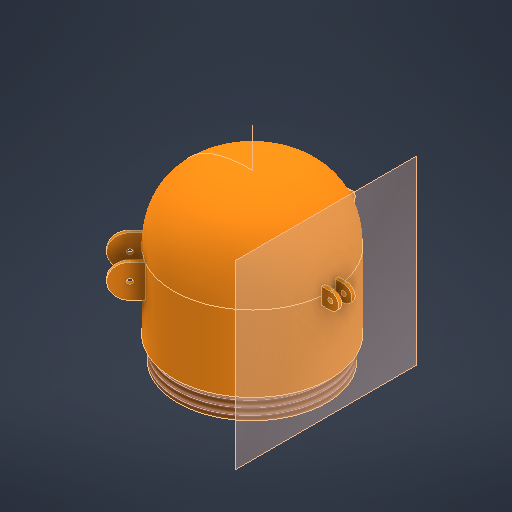
# Autodesk Inventor part: Head
Saved by Autodesk Inventor 2026.2 (Build 302298000, 298)
## iProperties
Created: 2026-06-05
Part Number: Head
Material: Generic
Document SubType Name: Modeling
Designer: User
Density: 1 g/cm^3
Appearance: Default
Author: User
Autodesk Inventor part; units mm, degrees
ref_plane "XZ Plane" through (0, 0, 0) normal (0, 1, 0) x (-1, 0, 0)
ref_plane "DiagPlane" through (0, 0, 0) normal (-0.7071068, 0, 0.7071068) x (0, -1, 0)
ref_plane "DiagPlane2" through (0, 0, 0) normal (0.7071068, 0, 0.7071068) x (0, 1, 0)
sketch "Sketch1" plane through (0, 0, 0) normal (0, 1, 0) x (-1, 0, 0)
  circle A0 centre (0, 0) radius 45
  circle A1 centre (0, 0) radius 43
  dimension "d0" = 90
  dimension "d1" = 2
  constraints: 2 centre point, 1 coincident
  measures "d0" diameter of A0
  measures "d1" radial gap between concentric circles of A0 A1
extrude "ThreadExtrude" add sketch "Sketch1" along normal blind 14
thread "Thread" size "M95x4" class "6g" standard "ANSI Metric M Profile" length 14.4
sketch "Sketch2" plane through (0, 14, 0) normal (0, 1, 0) x (1, 0, 0)
  circle A0 centre (0, 0) radius 47.5
  circle A1 centre (0, 0) radius 44
  dimension "d11" = 95
  dimension "d12" = 3.5
  constraints: 2 centre point, 2 coincident
  measures "d11" diameter of A0
  measures "d12" radial gap between concentric circles of A1 A0
extrude "FrontSideHead" add sketch "Sketch2" along normal blind 16
sketch "Sketch3" plane through (0, 0, 0) normal (0, 0, 1) x (1, 0, 0)
  line L0 (-32.31, 100) -> (33.2707, 100) construction
  line L1 (0, 100) -> (0, 30) construction
  line L2 (47.5, 30) -> (-47.5, 30) projected
  line L3 (-47.5, 30) -> (-47.5, 60)
  line L4 (-47.5, 60) -> (-47.5, 100) construction
  line L5 (-47.5, 100) -> (0, 100) construction
  spline S0 degree 2 poles (-47.5, 60) (-47.5, 100) (0, 100) knots 1 1 1 2 2 2
  line L6 (-44, 60) -> (-44, 32)
  line L7 (0, 96.5) -> (0, 100)
  line L8 (-44, 32) -> (-44, 30)
  line L9 (0, -22.4309) -> (0, 134.5853) projected
  spline S1 degree 5 poles (0, 96.5) (-4.007, 96.4999) (-8.0166, 96.3165) (-12.009, 95.9078) (-19.0004, 94.6845) (-25.6504, 92.2541) (-28.4308, 90.9379) (-33.3849, 87.8015) (-37.3693, 83.5133) (-38.9723, 81.2275) (-41.8114, 75.8309) (-43.3126, 69.9035) (-43.7834, 66.6139) (-44.0008, 63.3074) (-44, 60) knots 0 0 0 0 0 0 0.305355 0.305355 0.305355 0.538004 0.538004 0.538004 0.748006 0.748006 0.748006 1 1 1 1 1 1
  point P0 (0, 0)
  dimension "d21" = 3.5
  dimension "d19" = 40
  dimension "d20" = 30
  dimension "d22" = 0
  dimension "d23" = 2
  dimension "d24" = 33.2707
  dimension "d25" = 32.31
  constraints: 12 end point, 3 point on line, 3 vertical, 2 horizontal, 1 collinear, 1 parallel, 1 perpendicular, 6 other
  measures "d19" distance of L3.end L4.end
  measures "d20" distance of L2.end L3.end
  measures "d22" distance from line of L1.end L2
  measures "d23" distance from line of L6.end L2
  measures "d24" distance from line of L0.end L7
  measures "d25" distance from line of L0.start L7
revolve "BackSideHead" add sketch "Sketch3" angle 360 about axis through (0, 0, 0) along (0, 1, 0) contours L2 L3 S0 L7 S1 L6 L8
sketch "Sketch7" plane through (0, 0, 0) normal (-0.7071068, 0, 0.7071068) x (0, -1, 0)
  line L0 (-60, 44) -> (-60, -44) projected
  line L1 (-40, 10) -> (-60, 10)
  line L2 (-60, 10) -> (-60, -10)
  line L3 (-60, -10) -> (-40, -10)
  line L4 (-40, -10) -> (-40, 10)
  line L5 (-40, 10) -> (-60, -10) construction
  line L6 (-60, 10) -> (-40, -10) construction
  point P0 (0, 0)
  point P1 (-60, -31.1127)
  point P2 (-50, 0)
  dimension "d32" = 20
  constraints: 12 end point, 2 midpoint, 2 parallel, 2 perpendicular, 1 horizontal, 1 horizontal alignment, 1 point on line
  measures "d32" distance of L3.end L1.start
extrude "CableHole" cut sketch "Sketch7" along normal up to next
fillet "Fillet1" radius 3 4 edges at (-24.4956, 60, 38.6377) (-38.6377, 60, 24.4956) (-38.6377, 40, 24.4956) (-24.4956, 40, 38.6377)
ref_plane "BottomPlane" through (-33.5876, 60, 33.5876) normal (-0.7071068, 0, 0.7071068) x (0, -1, 0)
ref_plane "LeftEarPlane" through (0, 14, -47.5) normal (0, 0, 1) x (1, 0, 0)
ref_plane "RightEarPlane" through (47.5, 14, 0) normal (1, 0, 0) x (0, 1, 0)
sketch "Sketch13" plane through (-33.5876, 60, 33.5876) normal (-0.7071068, 0, 0.7071068) x (0, -1, 0)
  line L0 (0, -12) -> (20, -12)
  line L1 (20, -12) -> (20, -10)
  line L2 (20, -10) -> (0, -10)
  line L3 (0, -10) -> (0, -12)
  line L4 (0, -12) -> (20, -10) construction
  line L5 (20, -12) -> (0, -10) construction
  line L6 (17, -10) -> (3, -10) projected
  line L7 (20, -7) -> (20, 7) projected
  line L8 (0, 7) -> (0, -7) projected
  point P0 (60, 0)
  point P1 (10, -11)
  dimension "d39" = 2
  constraints: 12 end point, 3 collinear, 2 midpoint, 2 parallel, 1 horizontal, 1 perpendicular
  measures "d39" distance of L0.end L1.end
extrude "PitchAxisBase" add sketch "Sketch13" against normal up to surface round surface about axis through (0, 14, 0) along (0, 1, 0) radius 47.5 far side no
sketch "Sketch14" plane through (-42.0729, 40, 25.1023) normal (-0.7071068, 0, -0.7071068) x (-0.7071068, 0, 0.7071068)
  line L0 (0, 0) -> (0, 20) projected
  line L1 (0, 20) -> (5, 20)
  line L2 (0, 0) -> (5, 0)
  arc A0 (5, 0) -> (5, 20) centre (5, 10) ccw
  circle A1 centre (5, 10) radius 1.5
  point P0 (-47.5, -40)
  dimension "d42" = 5
  dimension "d45" = 3
  constraints: 4 end point, 2 centre point, 2 horizontal, 2 point on circle, 1 coincident, 1 parallel, 1 tangent
  measures "d42" distance from line of L0 A0.centre
  measures "d45" diameter of A1
extrude "PitchAxisHole" add sketch "Sketch14" against normal blind 2
mirror "PitchAxisHoleMirror" about plane through (0, 0, 0) normal (0.7071068, 0, 0.7071068) of "PitchAxisHole", "PitchAxisBase"
sketch "Sketch15" plane through (47.5, 14, 0) normal (1, 0, 0) x (0, 1, 0)
  line L0 (51, -5) -> (41, -5) construction
  line L1 (41, -5) -> (41, 5) construction
  line L2 (41, 5) -> (51, 5) construction
  line L3 (51, 5) -> (51, -5) construction
  line L4 (51, -5) -> (41, 5) construction
  line L5 (41, -5) -> (51, 5) construction
  line L6 (-34, 0) -> (106, 0) projected
  line L7 (46, -47.5) -> (46, 47.5) projected
  line L8 (51, 5) -> (41, 5)
  line L9 (41, 5) -> (41, 3)
  line L10 (41, 3) -> (51, 3)
  line L11 (51, 3) -> (51, 5)
  point P0 (-14, 0)
  point P1 (46, 0)
  point P2 (46, 40.9834)
  point P3 (46, 0)
  dimension "d46" = 10
  dimension "d47" = 2
  constraints: 20 end point, 4 parallel, 3 midpoint, 3 perpendicular, 2 horizontal, 2 point on line
  measures "d46" distance of L0.end L1.end
  measures "d47" distance between parallel lines of L10 L2
extrude "Extrusion8" add sketch "Sketch15" against normal up to surface round surface about axis through (0, 14, 0) along (0, 1, 0) radius 47.5 far side no
sketch "Sketch16" plane through (47.5, 55, 5) normal (0, 0, 1) x (1, 0, 0)
  line L0 (0, 0) -> (5.0003, 0)
  line L1 (0, 10) -> (0, 0) projected
  line L2 (0, 10) -> (5.0003, 10)
  arc A0 (5.0003, 0) -> (5.0003, 10) centre (5.0003, 5) ccw
  circle A1 centre (5.0003, 5) radius 1.5
  point P0 (-47.5, -55)
  dimension "d50" = 5.0003
  dimension "d51" = 3
  constraints: 4 end point, 2 centre point, 2 horizontal, 2 point on circle, 1 coincident, 1 parallel, 1 tangent
  measures "d50" distance from line of L1 A0.centre
  measures "d51" diameter of A1
extrude "Extrusion9" add sketch "Sketch16" against normal blind 2
mirror "Mirror2" about plane through (0, 0, 0) normal (0, 0, 1) of "Extrusion9", "Extrusion8"
mirror "Mirror3" about plane through (0, 0, 0) normal (0.7071068, 0, 0.7071068) of "Extrusion8", "Mirror2", "Extrusion9"
body "Solid1"
